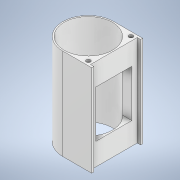
# Autodesk Inventor part: Tubo
Saved by Autodesk Inventor 2020.3 (Build 243373000, 373)
## iProperties
Created: 2020-07-24
Part Number: Tubo
Material: ABS Plastic
Document SubType Name: Modeling
Designer: juanp
Density: 1.06 g/cm^3
Appearance: Smooth - White
Author: juanp
Autodesk Inventor part; units mm, degrees
ref_plane "YZ Plane" through (0, 0, 0) normal (1, 0, 0) x (0, 1, 0)
ref_plane "XZ Plane" through (0, 0, 0) normal (0, 1, 0) x (-1, 0, 0)
ref_plane "XY Plane" through (0, 0, 0) normal (0, 0, 1) x (1, 0, 0)
sketch "Sketch1" plane through (0, 0, 0) normal (0, 1, 0) x (-1, 0, 0)
  circle A0 centre (0, 0) radius 18
  arc A1 (19, 0) -> (0, -19) centre (0, 0) ccw
  line L0 (19, -19) -> (0, -19) construction
  line L1 (-19, -19) -> (-19, 19)
  line L2 (-19, 19) -> (0, 19)
  line L3 (19, 19) -> (19, 0) construction
  line L4 (19, -19) -> (-19, 19) construction
  line L5 (-19, -19) -> (19, 19) construction
  line L6 (0, -19) -> (-19, -19)
  line L7 (19, 0) -> (19, -19) construction
  arc A2 (13.435, -13.435) -> (19, 0) centre (0, 0) ccw
  arc A3 (0, -19) -> (13.435, -13.435) centre (0, 0) ccw
  line L8 (0, 19) -> (19, 19) construction
  dimension "d0" = 36
  dimension "d1" = 38
  constraints: 18 end point, 7 point on circle, 6 parallel, 6 tangent, 4 centre point, 2 coincident, 2 horizontal, 2 midpoint, 2 perpendicular, 1 point on line
  measures "d0" diameter of A0
  measures "d1" diameter of A1
extrude "Extrusion1" add sketch "Sketch1" along normal blind 68
ref_plane "Work Plane2" through (0, 34, 0) normal (0, -1, 0) x (1, 0, 0)
sketch "Sketch10" plane through (0, 68, 0) normal (0, 1, 0) x (1, 0, 0)
  line L0 (19, -19) -> (19, 19) projected
  line L1 (19, 19) -> (12.7279, 12.7279) construction
  circle A0 centre (0, 0) radius 18 projected
  line L2 (0, -19) -> (19, -19) projected
  line L3 (19, -19) -> (12.7279, -12.7279) construction
  circle A1 centre (15.864, 15.864) radius 1.55
  circle A2 centre (15.864, -15.864) radius 1.55
  dimension "d21" = 3.1
  dimension "d22" = 3.1
  constraints: 4 end point, 2 centre point, 2 line through centre, 2 midpoint, 2 point on circle
  measures "d21" diameter of A1
  measures "d22" diameter of A2
extrude "Extrusion5" cut sketch "Sketch10" against normal through all contours A1 | A2
sketch "Sketch11" plane through (19, 0, 19) normal (1, 0, 0) x (0, 0, -1)
  line L0 (0, 68) -> (38, 68) projected
  line L1 (0, 0) -> (38, 0) projected
  line L2 (0, 68) -> (38, 0) construction
  line L3 (38, 68) -> (0, 0) construction
  line L4 (36.414, 68) -> (36.414, 0) projected
  line L5 (1.586, 51.5) -> (36.414, 51.5)
  line L6 (36.414, 51.5) -> (36.414, 16.5)
  line L7 (36.414, 16.5) -> (1.586, 16.5)
  line L8 (1.586, 16.5) -> (1.586, 51.5)
  line L9 (1.586, 51.5) -> (36.414, 16.5) construction
  line L10 (36.414, 51.5) -> (1.586, 16.5) construction
  point P0 (19, 0)
  point P1 (19, 34)
  dimension "d25" = 35
  constraints: 16 end point, 3 midpoint, 2 parallel, 1 horizontal, 1 perpendicular, 1 point on line
  measures "d25" distance of L5.end L6.end
extrude "Extrusion6" cut sketch "Sketch11" against normal up to next
sketch "Sketch12" plane through (19, 0, 19) normal (1, 0, 0) x (0, 0, -1)
  line L0 (0, 0) -> (0, 68) projected
  line L1 (1.586, 68) -> (4.686, 68) projected
  line L2 (0, 0) -> (1.586, 0)
  line L3 (1.586, 0) -> (1.586, 68)
  line L4 (1.586, 68) -> (0, 68)
  line L5 (0, 68) -> (0, 0)
  line L6 (0, 0) -> (38, 0) projected
  line L7 (36.414, 68) -> (36.414, 51.5) projected
  line L8 (38, 0) -> (36.414, 0)
  line L9 (36.414, 0) -> (36.414, 68)
  line L10 (36.414, 68) -> (38, 68)
  line L11 (38, 68) -> (38, 0)
  point P0 (19, 0)
  point P1 (0, 68)
  constraints: 16 end point, 4 parallel, 2 horizontal, 2 perpendicular, 2 point on line
extrude "Extrusion7" add sketch "Sketch12" along normal blind 2.5
sketch "Sketch13" plane through (19, 16.5, 17.414) normal (0, 1, 0) x (1, 0, 0)
  line L0 (0, 34.8279) -> (0, 0) projected
  line L1 (0, 34.8279) -> (-3.136, 34.8279) projected
  line L2 (-3.136, 34.8279) -> (-14.4443, 34.8279) projected
  arc A0 (-14.4443, 0) -> (-14.4443, 34.8279) centre (-19, 17.414) ccw projected
  circle A1 centre (-3.136, 33.2779) radius 1.55 projected
  circle A2 centre (-3.136, 33.2779) radius 1.55
  circle A3 centre (-3.136, 33.2779) radius 2.5 construction
  line L3 (0, 30.7779) -> (-6.9416, 30.7779)
  circle A4 centre (-19, 17.414) radius 18
  line L4 (0, 34.8279) -> (-14.4443, 34.8279)
  line L5 (0, 34.8279) -> (0, 30.7779)
  line L6 (-19, 17.414) -> (-15.9745, 17.414) construction
  line L7 (0, 0) -> (-3.136, 0)
  line L8 (-3.136, 0) -> (-14.4443, 0)
  circle A5 centre (-3.136, 1.55) radius 1.55
  circle A6 centre (-3.136, 1.55) radius 1.55
  circle A7 centre (-3.136, 1.55) radius 2.5 construction
  line L9 (0, 4.05) -> (-6.9416, 4.05)
  line L10 (0, 0) -> (-14.4443, 0)
  line L11 (0, 0) -> (0, 4.05)
  point P0 (0, 4.05)
  point P1 (-6.9416, 4.05)
  dimension "d30" = 5
  constraints: 18 end point, 6 symmetric about line, 5 centre point, 5 coincident, 3 horizontal, 2 vertical alignment, 1 collinear, 1 concentric, 1 perpendicular, 1 point on circle, 1 point on line, 1 tangent, 4 other
  measures "d30" diameter of A3
extrude "Extrusion8" add sketch "Sketch13" along normal up to next contours L0 L3 A0 L2 L1 | L0 L7 L8 A0 L9
body "Solid1"
